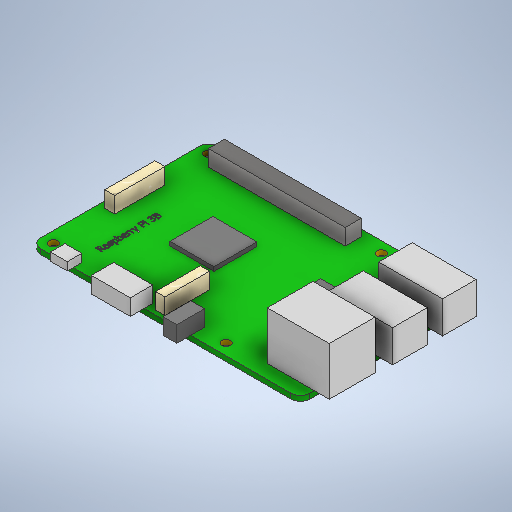
# Autodesk Inventor part: RPi3B
Saved by Autodesk Inventor 2025 (Build 290162000, 162)
## iProperties
Created: 2025-05-10
Part Number: RPi3B
Material: Generic
Document SubType Name: Modeling
Designer: thesn
Density: 1 g/cm^3
Appearance: Default
Author: thesn
Autodesk Inventor part; units mm, degrees
ref_plane "YZ Plane" through (0, 0, 0) normal (1, 0, 0) x (0, 1, 0)
ref_plane "XZ Plane" through (0, 0, 0) normal (0, 1, 0) x (-1, 0, 0)
ref_plane "XY Plane" through (0, 0, 0) normal (0, 0, 1) x (1, 0, 0)
sketch "Sketch1" plane through (0, 0, 0) normal (0, 1, 0) x (-1, 0, 0)
  line L0 (0, 0) -> (-85.0001, 0)
  line L1 (-85.0001, 0) -> (-85.0001, -55.9999)
  line L2 (-85.0001, -55.9999) -> (0, -55.9999)
  line L3 (0, -55.9999) -> (0, 0)
  dimension "d0" = 85.0001
  dimension "d1" = 55.9999
  constraints: 8 end point, 2 parallel, 1 horizontal, 1 perpendicular
  measures "d0" distance of L2.end L1.end
  measures "d1" distance of L1.end L0.end
extrude "Extrusion1" add sketch "Sketch1" along normal blind 1.6
fillet "Fillet1" radius 3 4 edges at (0, 0.8, -55.9999) (85.0001, 0.8, -55.9999) (0, 0.8, 0) (85.0001, 0.8, 0)
sketch "Sketch2" plane through (0, 1.6, 0) normal (0, 1, 0) x (1, 0, 0)
  circle A0 centre (3.5, 3.5) radius 1.375
  line L0 (3, 0) -> (82.0001, 0) projected
  line L1 (0, 52.9999) -> (0, 3) projected
  circle A1 centre (3.5, 52.4999) radius 1.375
  circle A2 centre (58.0001, 52.4999) radius 1.375
  circle A3 centre (58.0001, 3.5) radius 1.375
  line L2 (82.0001, 55.9999) -> (3, 55.9999) projected
  line L3 (85.0001, 3) -> (85.0001, 52.9999) projected
  point P0 (0, 0)
  dimension "d5" = 2.75
  dimension "d6" = 3.5
  dimension "d7" = 3.5
  dimension "d10" = 2.75
  dimension "d11" = 2.75
  dimension "d12" = 2.75
  dimension "d13" = 3.5
  dimension "d14" = 3.5
  dimension "d15" = 3.5
  dimension "d16" = 3.5
  dimension "d17" = 26.9999
  dimension "d18" = 26.9999
  constraints: 4 centre point
  measures "d5" diameter of A0
  measures "d6" distance from line of L0 A0.centre
  measures "d7" distance from line of L1 A0.centre
  measures "d10" diameter of A1
  measures "d11" diameter of A2
  measures "d12" diameter of A3
  measures "d13" distance from line of L1 A1.centre
  measures "d14" distance from line of L2 A1.centre
  measures "d15" distance from line of L2 A2.centre
  measures "d16" distance from line of L0 A3.centre
  measures "d17" distance from line of L3 A2.centre
  measures "d18" distance from line of L3 A3.centre
extrude "Extrusion2" cut sketch "Sketch2" against normal blind 25.4
sketch "Sketch3" plane through (0, 1.6, 0) normal (0, 1, 0) x (1, 0, 0)
  line L0 (7.1379, 53.8738) -> (50.3179, 53.8738)
  line L1 (50.3179, 53.8738) -> (50.3179, 48.7938)
  line L2 (50.3179, 48.7938) -> (7.1379, 48.7938)
  line L3 (7.1379, 48.7938) -> (7.1379, 53.8738)
  line L4 (70.1256, 50.1514) -> (90.2699, 50.1514)
  line L5 (90.2699, 50.1514) -> (90.2699, 39.5684)
  line L6 (90.2699, 39.5684) -> (70.1256, 39.5684)
  line L7 (70.1256, 39.5684) -> (70.1256, 50.1514)
  line L8 (70.1256, 34.7512) -> (90.2699, 34.7512)
  line L9 (90.2699, 34.7512) -> (90.2699, 23.8032)
  line L10 (90.2699, 23.8032) -> (70.1256, 23.8032)
  line L11 (70.1256, 23.8032) -> (70.1256, 34.7512)
  line L12 (70.1256, 18.8401) -> (89.686, 18.8401)
  line L13 (89.686, 18.8401) -> (89.686, 4.3887)
  line L14 (89.686, 4.3887) -> (70.1256, 4.3887)
  line L15 (70.1256, 4.3887) -> (70.1256, 18.8401)
  line L16 (7.9408, 2.71) -> (13.2688, 2.71)
  line L17 (13.2688, 2.71) -> (13.2688, -1.8882)
  line L18 (13.2688, -1.8882) -> (7.9408, -1.8882)
  line L19 (7.9408, -1.8882) -> (7.9408, 2.71)
  line L20 (23.3149, 2.71) -> (35.6326, 2.71)
  line L21 (35.6326, 2.71) -> (35.6326, -4.3596)
  line L22 (35.6326, -4.3596) -> (23.3149, -4.3596)
  line L23 (23.3149, -4.3596) -> (23.3149, 2.71)
  line L24 (45.9794, 4.3887) -> (50.3179, 4.3887)
  line L25 (50.3179, 4.3887) -> (50.3179, -4.3596)
  line L26 (50.3179, -4.3596) -> (45.9794, -4.3596)
  line L27 (45.9794, -4.3596) -> (45.9794, 4.3887)
  line L28 (2.0299, 37.0278) -> (5.1833, 37.0278)
  line L29 (5.1833, 37.0278) -> (5.1833, 21.1626)
  line L30 (5.1833, 21.1626) -> (2.0299, 21.1626)
  line L31 (2.0299, 21.1626) -> (2.0299, 37.0278)
  line L32 (22.6251, 34.7512) -> (36.5195, 34.7512)
  line L33 (36.5195, 34.7512) -> (36.5195, 21.1626)
  line L34 (36.5195, 21.1626) -> (22.6251, 21.1626)
  line L35 (22.6251, 21.1626) -> (22.6251, 34.7512)
  line L36 (56.6219, 34.7512) -> (65.4907, 34.7512)
  line L37 (65.4907, 34.7512) -> (65.4907, 26.0897)
  line L38 (65.4907, 26.0897) -> (56.6219, 26.0897)
  line L39 (56.6219, 26.0897) -> (56.6219, 34.7512)
  line L40 (37.899, 15.4472) -> (40.8553, 15.4472)
  line L41 (40.8553, 15.4472) -> (40.8553, 1.3558)
  line L42 (40.8553, 1.3558) -> (37.899, 1.3558)
  line L43 (37.899, 1.3558) -> (37.899, 15.4472)
  point P0 (0, 0)
  dimension "d19" = 43.18
  dimension "d20" = 5.08
  constraints: 88 end point, 22 parallel, 11 horizontal, 11 perpendicular, 9 point on line
  measures "d19" distance of L1.end L2.end
  measures "d20" distance of L0.end L1.end
extrude "Extrusion3" add sketch "Sketch3" along normal blind 10.16 contours L4 L5 L6 L7 | L8 L9 L10 L11
extrude "Extrusion4" add sketch "Sketch3" along normal blind 15.24 contours L12 L13 L14 L15
extrude "Extrusion5" add sketch "Sketch3" along normal blind 5.08 contours L0 L1 L2 L3
extrude "Extrusion6" add sketch "Sketch3" along normal blind 1.27 contours L32 L33 L34 L35 | L36 L37 L38 L39
extrude "Extrusion7" add sketch "Sketch3" along normal blind 5.08 contours L28 L29 L30 L31 | L40 L41 L42 L43
extrude "Extrusion8" add sketch "Sketch3" along normal blind 5.08 contours L20 L21 L22 L23
extrude "Extrusion9" add sketch "Sketch3" along normal blind 2.54 contours L16 L17 L18 L19
extrude "Extrusion10" add sketch "Sketch3" along normal blind 5.08 contours L24 L25 L26 L27
sketch "Sketch4" plane through (0, 0, 0) normal (0, -1, 0) x (1, 0, 0)
  line L0 (28.4319, -19.6331) -> (43.4029, -19.6331)
  line L1 (43.4029, -19.6331) -> (43.4029, -33.6849)
  line L2 (43.4029, -33.6849) -> (28.4319, -33.6849)
  line L3 (28.4319, -33.6849) -> (28.4319, -19.6331)
  line L4 (0.8536, -19.6331) -> (8.7331, -19.6331)
  line L5 (8.7331, -19.6331) -> (8.7331, -30.2704)
  line L6 (8.7331, -30.2704) -> (0.8536, -30.2704)
  line L7 (0.8536, -30.2704) -> (0.8536, -19.6331)
  point P0 (0, 0)
  constraints: 16 end point, 4 parallel, 2 horizontal, 2 perpendicular, 1 point on line
extrude "Extrusion11" add sketch "Sketch4" along normal blind 1.27 contours L0 L1 L2 L3
extrude "Extrusion12" add sketch "Sketch4" along normal blind 0.508 contours L4 L5 L6 L7
sketch "Sketch5" plane through (0, 1.6, 0) normal (0, 1, 0) x (1, 0, 0)
  line L0 (11.2333, 8.619) -> (11.2333, 37.8862) construction
  line L1 (11.2333, 37.8862) -> (15.2594, 37.8862) construction
  line L2 (15.2594, 37.8862) -> (15.2594, 8.619) construction
  line L3 (15.2594, 8.619) -> (11.2333, 8.619) construction
  line L4 (13.3559, 10.3974) -> (13.3559, 10.0467)
  line L5 (13.3559, 10.0467) -> (12.5474, 9.4045)
  line L6 (12.5474, 9.4045) -> (12.5474, 9.0949)
  line L7 (12.5474, 9.0949) -> (13.3559, 9.0949)
  line L8 (13.3559, 9.0949) -> (13.3559, 8.8249)
  line L9 (13.3559, 8.8249) -> (11.3239, 8.8249)
  line L10 (11.3239, 8.8249) -> (11.3239, 9.3485)
  spline S0 degree 2 poles (11.3239, 9.3485) (11.3239, 9.523) (11.3618, 9.7585) (11.4309, 9.8656) knots 0 0 0 1 2 2 2
  spline S1 degree 2 poles (11.4309, 9.8656) (11.5001, 9.9726) (11.7158, 10.0961) (11.8755, 10.0961) knots 0 0 0 1 2 2 2
  spline S2 degree 2 poles (11.8755, 10.0961) (12.0978, 10.0961) (12.3992, 9.8688) (12.4716, 9.6745) knots 0 0 0 1 2 2 2
  line L11 (12.4716, 9.6745) -> (13.3559, 10.3974)
  spline S3 degree 2 poles (11.8969, 9.8145) (11.808, 9.8145) (11.6713, 9.7519) (11.6269, 9.6861) knots 0 0 0 1 2 2 2
  spline S4 degree 2 poles (11.6269, 9.6861) (11.589, 9.6284) (11.5577, 9.4753) (11.5577, 9.3633) knots 0 0 0 1 2 2 2
  line L12 (11.5577, 9.3633) -> (11.5577, 9.0949)
  line L13 (11.5577, 9.0949) -> (12.3218, 9.0949)
  line L14 (12.3218, 9.0949) -> (12.3218, 9.332)
  spline S5 degree 2 poles (12.3218, 9.332) (12.3218, 9.4489) (12.2806, 9.635) (12.2164, 9.6992) knots 0 0 0 1 2 2 2
  spline S6 degree 2 poles (12.2164, 9.6992) (12.1604, 9.7585) (12.0023, 9.8145) (11.8969, 9.8145) knots 0 0 0 1 2 2 2
  spline S7 degree 2 poles (13.1945, 11.3887) (13.2176, 11.3574) (13.2999, 11.2521) (13.3246, 11.2027) knots 0 0 0 1 2 2 2
  spline S8 degree 2 poles (13.3246, 11.2027) (13.3608, 11.1351) (13.3987, 11.0083) (13.3987, 10.8931) knots 0 0 0 1 2 2 2
  spline S9 degree 2 poles (13.3987, 10.8931) (13.3987, 10.7992) (13.3279, 10.6296) (13.2637, 10.5654) knots 0 0 0 1 2 2 2
  spline S10 degree 2 poles (13.2637, 10.5654) (13.2011, 10.5045) (13.0167, 10.4304) (12.9146, 10.4304) knots 0 0 0 1 2 2 2
  spline S11 degree 2 poles (12.9146, 10.4304) (12.7565, 10.4304) (12.5325, 10.5637) (12.4683, 10.7087) knots 0 0 0 1 2 2 2
  spline S12 degree 2 poles (12.4683, 10.7087) (12.409, 10.8371) (12.3646, 11.1862) (12.3531, 11.3887) knots 0 0 0 1 2 2 2
  line L15 (12.3531, 11.3887) -> (12.3037, 11.3887)
  spline S13 degree 2 poles (12.3037, 11.3887) (12.2147, 11.3887) (12.1044, 11.3344) (12.0731, 11.285) knots 0 0 0 1 2 2 2
  spline S14 degree 2 poles (12.0731, 11.285) (12.0418, 11.2356) (12.0221, 11.094) (12.0221, 11.0182) knots 0 0 0 1 2 2 2
  spline S15 degree 2 poles (12.0221, 11.0182) (12.0221, 10.9293) (12.0748, 10.6889) (12.1258, 10.5687) knots 0 0 0 1 2 2 2
  line L16 (12.1258, 10.5687) -> (12.1258, 10.5539)
  line L17 (12.1258, 10.5539) -> (11.864, 10.5539)
  spline S16 degree 2 poles (11.864, 10.5539) (11.8442, 10.6247) (11.7948, 10.8898) (11.7948, 11.0199) knots 0 0 0 1 2 2 2
  spline S17 degree 2 poles (11.7948, 11.0199) (11.7948, 11.178) (11.8442, 11.3937) (11.9085, 11.4793) knots 0 0 0 1 2 2 2
  spline S18 degree 2 poles (11.9085, 11.4793) (11.971, 11.5633) (12.1703, 11.6456) (12.3135, 11.6456) knots 0 0 0 1 2 2 2
  line L18 (12.3135, 11.6456) -> (13.3559, 11.6456)
  line L19 (13.3559, 11.6456) -> (13.3559, 11.3887)
  line L20 (13.3559, 11.3887) -> (13.1945, 11.3887)
  line L21 (12.9804, 11.3887) -> (12.5572, 11.3887)
  spline S19 degree 2 poles (12.5572, 11.3887) (12.5655, 11.2965) (12.5935, 11.0182) (12.6198, 10.931) knots 0 0 0 1 2 2 2
  spline S20 degree 2 poles (12.6198, 10.931) (12.6511, 10.8289) (12.7812, 10.6955) (12.8965, 10.6955) knots 0 0 0 1 2 2 2
  spline S21 degree 2 poles (12.8965, 10.6955) (13.0282, 10.6955) (13.1616, 10.8437) (13.1616, 10.9853) knots 0 0 0 1 2 2 2
  spline S22 degree 2 poles (13.1616, 10.9853) (13.1616, 11.1055) (13.0578, 11.3031) (12.9804, 11.3887) knots 0 0 0 1 2 2 2
  spline S23 degree 2 poles (13.3921, 12.4179) (13.3921, 12.2648) (13.3098, 11.9996) (13.2637, 11.9124) knots 0 0 0 1 2 2 2
  line L22 (13.2637, 11.9124) -> (12.9755, 11.9124)
  line L23 (12.9755, 11.9124) -> (12.9755, 11.9255)
  spline S24 degree 2 poles (12.9755, 11.9255) (13.0019, 11.9585) (13.0644, 12.0474) (13.099, 12.1215) knots 0 0 0 1 2 2 2
  spline S25 degree 2 poles (13.099, 12.1215) (13.1303, 12.1857) (13.1764, 12.3438) (13.1764, 12.4278) knots 0 0 0 1 2 2 2
  spline S26 degree 2 poles (13.1764, 12.4278) (13.1764, 12.4887) (13.1484, 12.6287) (13.1254, 12.6616) knots 0 0 0 1 2 2 2
  spline S27 degree 2 poles (13.1254, 12.6616) (13.0941, 12.7094) (13.0233, 12.7522) (12.9508, 12.7522) knots 0 0 0 1 2 2 2
  spline S28 degree 2 poles (12.9508, 12.7522) (12.8602, 12.7522) (12.7664, 12.6534) (12.7351, 12.5266) knots 0 0 0 1 2 2 2
  spline S29 degree 2 poles (12.7351, 12.5266) (12.7236, 12.4772) (12.6906, 12.3191) (12.6725, 12.2516) knots 0 0 0 1 2 2 2
  spline S30 degree 2 poles (12.6725, 12.2516) (12.6215, 12.077) (12.4107, 11.919) (12.2608, 11.919) knots 0 0 0 1 2 2 2
  spline S31 degree 2 poles (12.2608, 11.919) (12.0534, 11.919) (11.7948, 12.2302) (11.7948, 12.4871) knots 0 0 0 1 2 2 2
  spline S32 degree 2 poles (11.7948, 12.4871) (11.7948, 12.6139) (11.8574, 12.8707) (11.9052, 12.958) knots 0 0 0 1 2 2 2
  line L24 (11.9052, 12.958) -> (12.1802, 12.958)
  line L25 (12.1802, 12.958) -> (12.1802, 12.9448)
  spline S33 degree 2 poles (12.1802, 12.9448) (12.1011, 12.846) (12.0106, 12.6056) (12.0106, 12.4821) knots 0 0 0 1 2 2 2
  spline S34 degree 2 poles (12.0106, 12.4821) (12.0106, 12.3553) (12.1176, 12.1808) (12.2246, 12.1808) knots 0 0 0 1 2 2 2
  spline S35 degree 2 poles (12.2246, 12.1808) (12.3218, 12.1808) (12.4156, 12.2845) (12.4453, 12.3998) knots 0 0 0 1 2 2 2
  spline S36 degree 2 poles (12.4453, 12.3998) (12.4601, 12.4558) (12.4897, 12.5974) (12.5078, 12.6748) knots 0 0 0 1 2 2 2
  spline S37 degree 2 poles (12.5078, 12.6748) (12.5507, 12.8427) (12.7466, 13.014) (12.9162, 13.014) knots 0 0 0 1 2 2 2
  spline S38 degree 2 poles (12.9162, 13.014) (13.015, 13.014) (13.1896, 12.9366) (13.2538, 12.8609) knots 0 0 0 1 2 2 2
  spline S39 degree 2 poles (13.2538, 12.8609) (13.3213, 12.7802) (13.3921, 12.5743) (13.3921, 12.4179) knots 0 0 0 1 2 2 2
  spline S40 degree 2 poles (12.5523, 14.5306) (12.9343, 14.5306) (13.3855, 14.1667) (13.3855, 13.8884) knots 0 0 0 1 2 2 2
  spline S41 degree 2 poles (13.3855, 13.8884) (13.3855, 13.7748) (13.3328, 13.6002) (13.2785, 13.5097) knots 0 0 0 1 2 2 2
  line L26 (13.2785, 13.5097) -> (13.9174, 13.5097)
  line L27 (13.9174, 13.5097) -> (13.9174, 13.2528)
  line L28 (13.9174, 13.2528) -> (11.8311, 13.2528)
  line L29 (11.8311, 13.2528) -> (11.8311, 13.5097)
  line L30 (11.8311, 13.5097) -> (11.9908, 13.5097)
  spline S42 degree 2 poles (11.9908, 13.5097) (11.9035, 13.6052) (11.7882, 13.839) (11.7882, 13.9757) knots 0 0 0 1 2 2 2
  spline S43 degree 2 poles (11.7882, 13.9757) (11.7882, 14.2375) (12.2032, 14.5306) (12.5523, 14.5306) knots 0 0 0 1 2 2 2
  spline S44 degree 2 poles (12.5819, 14.2655) (12.3201, 14.2655) (12.032, 14.0992) (12.032, 13.9131) knots 0 0 0 1 2 2 2
  spline S45 degree 2 poles (12.032, 13.9131) (12.032, 13.8044) (12.1291, 13.6002) (12.2049, 13.5097) knots 0 0 0 1 2 2 2
  line L31 (12.2049, 13.5097) -> (13.071, 13.5097)
  spline S46 degree 2 poles (13.071, 13.5097) (13.1188, 13.6101) (13.155, 13.7534) (13.155, 13.8456) knots 0 0 0 1 2 2 2
  spline S47 degree 2 poles (13.155, 13.8456) (13.155, 14.0448) (12.8619, 14.2655) (12.5819, 14.2655) knots 0 0 0 1 2 2 2
  spline S48 degree 2 poles (12.5688, 16.0752) (12.9426, 16.0752) (13.3987, 15.7129) (13.3987, 15.4396) knots 0 0 0 1 2 2 2
  spline S49 degree 2 poles (13.3987, 15.4396) (13.3987, 15.3161) (13.3378, 15.1399) (13.2851, 15.0542) knots 0 0 0 1 2 2 2
  line L32 (13.2851, 15.0542) -> (13.3559, 15.0378)
  line L33 (13.3559, 15.0378) -> (13.3559, 14.7974)
  line L34 (13.3559, 14.7974) -> (11.2333, 14.7974)
  line L35 (11.2333, 14.7974) -> (11.2333, 15.0542)
  line L36 (11.2333, 15.0542) -> (11.9908, 15.0542)
  spline S50 degree 2 poles (11.9908, 15.0542) (11.9035, 15.1514) (11.7882, 15.377) (11.7882, 15.5202) knots 0 0 0 1 2 2 2
  spline S51 degree 2 poles (11.7882, 15.5202) (11.7882, 15.7788) (12.2016, 16.0752) (12.5688, 16.0752) knots 0 0 0 1 2 2 2
  spline S52 degree 2 poles (12.5885, 15.8101) (12.3152, 15.8101) (12.032, 15.6437) (12.032, 15.4593) knots 0 0 0 1 2 2 2
  spline S53 degree 2 poles (12.032, 15.4593) (12.032, 15.3556) (12.1308, 15.1415) (12.2065, 15.0542) knots 0 0 0 1 2 2 2
  line L37 (12.2065, 15.0542) -> (13.0809, 15.0542)
  spline S54 degree 2 poles (13.0809, 15.0542) (13.1286, 15.1514) (13.1682, 15.3012) (13.1682, 15.3902) knots 0 0 0 1 2 2 2
  spline S55 degree 2 poles (13.1682, 15.3902) (13.1682, 15.5861) (12.8899, 15.8101) (12.5885, 15.8101) knots 0 0 0 1 2 2 2
  spline S56 degree 2 poles (13.3905, 17.0039) (13.3905, 16.6383) (12.9804, 16.2366) (12.6017, 16.2366) knots 0 0 0 1 2 2 2
  spline S57 degree 2 poles (12.6017, 16.2366) (12.2296, 16.2366) (11.7882, 16.6268) (11.7882, 16.9413) knots 0 0 0 1 2 2 2
  spline S58 degree 2 poles (11.7882, 16.9413) (11.7882, 17.0829) (11.8706, 17.302) (11.9579, 17.3826) knots 0 0 0 1 2 2 2
  spline S59 degree 2 poles (11.9579, 17.3826) (12.0451, 17.465) (12.2971, 17.5522) (12.4799, 17.5522) knots 0 0 0 1 2 2 2
  line L38 (12.4799, 17.5522) -> (12.6198, 17.5522)
  line L39 (12.6198, 17.5522) -> (12.6198, 16.4967)
  spline S60 degree 2 poles (12.6198, 16.4967) (12.8849, 16.4967) (13.1665, 16.7635) (13.1665, 17.0006) knots 0 0 0 1 2 2 2
  spline S61 degree 2 poles (13.1665, 17.0006) (13.1665, 17.0846) (13.1286, 17.2476) (13.099, 17.3135) knots 0 0 0 1 2 2 2
  spline S62 degree 2 poles (13.099, 17.3135) (13.0661, 17.3826) (13.0084, 17.4781) (12.9821, 17.5094) knots 0 0 0 1 2 2 2
  line L40 (12.9821, 17.5094) -> (12.9821, 17.5243)
  line L41 (12.9821, 17.5243) -> (13.262, 17.5243)
  spline S63 degree 2 poles (13.262, 17.5243) (13.2801, 17.4798) (13.3328, 17.3448) (13.3477, 17.2921) knots 0 0 0 1 2 2 2
  spline S64 degree 2 poles (13.3477, 17.2921) (13.3691, 17.218) (13.3905, 17.0961) (13.3905, 17.0039) knots 0 0 0 1 2 2 2
  spline S65 degree 2 poles (12.4239, 17.302) (12.3201, 17.2987) (12.1686, 17.2558) (12.1176, 17.2147) knots 0 0 0 1 2 2 2
  spline S66 degree 2 poles (12.1176, 17.2147) (12.06, 17.1702) (11.999, 17.0302) (11.999, 16.9265) knots 0 0 0 1 2 2 2
  spline S67 degree 2 poles (11.999, 16.9265) (11.999, 16.8244) (12.06, 16.6812) (12.1192, 16.6219) knots 0 0 0 1 2 2 2
  spline S68 degree 2 poles (12.1192, 16.6219) (12.1802, 16.5642) (12.3267, 16.505) (12.4239, 16.4967) knots 0 0 0 1 2 2 2
  line L42 (12.4239, 16.4967) -> (12.4239, 17.302)
  line L43 (12.1061, 18.6209) -> (12.1061, 18.6078)
  spline S69 degree 2 poles (12.1061, 18.6078) (12.0978, 18.5781) (12.0945, 18.5139) (12.0945, 18.4694) knots 0 0 0 1 2 2 2
  spline S70 degree 2 poles (12.0945, 18.4694) (12.0945, 18.3657) (12.1851, 18.1615) (12.274, 18.0693) knots 0 0 0 1 2 2 2
  line L44 (12.274, 18.0693) -> (13.3559, 18.0693)
  line L45 (13.3559, 18.0693) -> (13.3559, 17.8124)
  line L46 (13.3559, 17.8124) -> (11.8311, 17.8124)
  line L47 (11.8311, 17.8124) -> (11.8311, 18.0693)
  line L48 (11.8311, 18.0693) -> (12.0583, 18.0693)
  spline S71 degree 2 poles (12.0583, 18.0693) (11.9332, 18.2093) (11.8311, 18.4184) (11.8311, 18.5172) knots 0 0 0 1 2 2 2
  spline S72 degree 2 poles (11.8311, 18.5172) (11.8311, 18.5567) (11.8344, 18.5962) (11.8393, 18.6209) knots 0 0 0 1 2 2 2
  line L49 (11.8393, 18.6209) -> (12.1061, 18.6209)
  line L50 (12.1061, 19.6287) -> (12.1061, 19.6155)
  spline S73 degree 2 poles (12.1061, 19.6155) (12.0978, 19.5859) (12.0945, 19.5217) (12.0945, 19.4772) knots 0 0 0 1 2 2 2
  spline S74 degree 2 poles (12.0945, 19.4772) (12.0945, 19.3735) (12.1851, 19.1693) (12.274, 19.0771) knots 0 0 0 1 2 2 2
  line L51 (12.274, 19.0771) -> (13.3559, 19.0771)
  line L52 (13.3559, 19.0771) -> (13.3559, 18.8202)
  line L53 (13.3559, 18.8202) -> (11.8311, 18.8202)
  line L54 (11.8311, 18.8202) -> (11.8311, 19.0771)
  line L55 (11.8311, 19.0771) -> (12.0583, 19.0771)
  spline S75 degree 2 poles (12.0583, 19.0771) (11.9332, 19.217) (11.8311, 19.4262) (11.8311, 19.525) knots 0 0 0 1 2 2 2
  spline S76 degree 2 poles (11.8311, 19.525) (11.8311, 19.5645) (11.8344, 19.604) (11.8393, 19.6287) knots 0 0 0 1 2 2 2
  line L56 (11.8393, 19.6287) -> (12.1061, 19.6287)
  line L57 (11.8311, 21.0251) -> (13.9174, 20.205)
  line L58 (13.9174, 20.205) -> (13.9174, 19.93)
  line L59 (13.9174, 19.93) -> (13.2818, 20.2034)
  line L60 (13.2818, 20.2034) -> (11.8311, 19.6501)
  line L61 (11.8311, 19.6501) -> (11.8311, 19.9268)
  line L62 (11.8311, 19.9268) -> (12.9607, 20.3434)
  line L63 (12.9607, 20.3434) -> (11.8311, 20.7583)
  line L64 (11.8311, 20.7583) -> (11.8311, 21.0251)
  spline S77 degree 2 poles (11.9365, 23.3963) (12.0682, 23.3963) (12.3053, 23.3024) (12.3876, 23.2185) knots 0 0 0 1 2 2 2
  spline S78 degree 2 poles (12.3876, 23.2185) (12.4914, 23.1131) (12.5984, 22.8282) (12.5984, 22.6108) knots 0 0 0 1 2 2 2
  line L65 (12.5984, 22.6108) -> (12.5984, 22.382)
  line L66 (12.5984, 22.382) -> (13.3559, 22.382)
  line L67 (13.3559, 22.382) -> (13.3559, 22.1119)
  line L68 (13.3559, 22.1119) -> (11.3239, 22.1119)
  line L69 (11.3239, 22.1119) -> (11.3239, 22.6224)
  spline S79 degree 2 poles (11.3239, 22.6224) (11.3239, 22.8035) (11.3832, 23.0571) (11.4507, 23.1542) knots 0 0 0 1 2 2 2
  spline S80 degree 2 poles (11.4507, 23.1542) (11.5281, 23.2679) (11.7668, 23.3963) (11.9365, 23.3963) knots 0 0 0 1 2 2 2
  spline S81 degree 2 poles (11.9447, 23.1147) (11.8393, 23.1147) (11.6845, 23.0423) (11.6351, 22.9682) knots 0 0 0 1 2 2 2
  spline S82 degree 2 poles (11.6351, 22.9682) (11.5923, 22.9039) (11.5577, 22.7327) (11.5577, 22.6059) knots 0 0 0 1 2 2 2
  line L70 (11.5577, 22.6059) -> (11.5577, 22.382)
  line L71 (11.5577, 22.382) -> (12.3679, 22.382)
  line L72 (12.3679, 22.382) -> (12.3679, 22.5664)
  spline S83 degree 2 poles (12.3679, 22.5664) (12.3679, 22.731) (12.3152, 22.9336) (12.246, 22.9995) knots 0 0 0 1 2 2 2
  spline S84 degree 2 poles (12.246, 22.9995) (12.1851, 23.0604) (12.0418, 23.1147) (11.9447, 23.1147) knots 0 0 0 1 2 2 2
  line L73 (13.3559, 23.8952) -> (13.3559, 23.6384)
  line L74 (13.3559, 23.6384) -> (11.8311, 23.6384)
  line L75 (11.8311, 23.6384) -> (11.8311, 23.8952)
  line L76 (11.8311, 23.8952) -> (13.3559, 23.8952)
  line L77 (11.5775, 23.9134) -> (11.5775, 23.6219)
  line L78 (11.5775, 23.6219) -> (11.3107, 23.6219)
  line L79 (11.3107, 23.6219) -> (11.3107, 23.9134)
  line L80 (11.3107, 23.9134) -> (11.5775, 23.9134)
  spline S85 degree 2 poles (11.5165, 25.6555) (11.5165, 25.5814) (11.5528, 25.4349) (11.5808, 25.3641) knots 0 0 0 1 2 2 2
  spline S86 degree 2 poles (11.5808, 25.3641) (11.6088, 25.2982) (11.668, 25.2011) (11.6944, 25.1632) knots 0 0 0 1 2 2 2
  line L81 (11.6944, 25.1632) -> (11.6944, 25.1467)
  line L82 (11.6944, 25.1467) -> (11.4062, 25.1467)
  spline S87 degree 2 poles (11.4062, 25.1467) (11.3585, 25.2356) (11.2811, 25.5403) (11.2811, 25.677) knots 0 0 0 1 2 2 2
  spline S88 degree 2 poles (11.2811, 25.677) (11.2811, 25.8153) (11.3371, 26.0211) (11.3963, 26.1051) knots 0 0 0 1 2 2 2
  spline S89 degree 2 poles (11.3963, 26.1051) (11.4606, 26.194) (11.6466, 26.2862) (11.7718, 26.2862) knots 0 0 0 1 2 2 2
  spline S90 degree 2 poles (11.7718, 26.2862) (11.9397, 26.2862) (12.1933, 26.0656) (12.2263, 25.9108) knots 0 0 0 1 2 2 2
  line L83 (12.2263, 25.9108) -> (12.246, 25.9108)
  spline S91 degree 2 poles (12.246, 25.9108) (12.2592, 25.975) (12.3185, 26.1216) (12.3778, 26.1841) knots 0 0 0 1 2 2 2
  spline S92 degree 2 poles (12.3778, 26.1841) (12.4354, 26.2467) (12.6198, 26.3257) (12.7532, 26.3257) knots 0 0 0 1 2 2 2
  spline S93 degree 2 poles (12.7532, 26.3257) (12.8899, 26.3257) (13.1221, 26.2319) (13.211, 26.1463) knots 0 0 0 1 2 2 2
  spline S94 degree 2 poles (13.211, 26.1463) (13.3032, 26.0573) (13.3987, 25.8054) (13.3987, 25.6457) knots 0 0 0 1 2 2 2
  spline S95 degree 2 poles (13.3987, 25.6457) (13.3987, 25.4925) (13.3246, 25.1928) (13.2736, 25.0907) knots 0 0 0 1 2 2 2
  line L84 (13.2736, 25.0907) -> (12.9854, 25.0907)
  line L85 (12.9854, 25.0907) -> (12.9854, 25.1105)
  spline S96 degree 2 poles (12.9854, 25.1105) (13.048, 25.1961) (13.1632, 25.4859) (13.1632, 25.6292) knots 0 0 0 1 2 2 2
  spline S97 degree 2 poles (13.1632, 25.6292) (13.1632, 25.7132) (13.1105, 25.8811) (13.0496, 25.9371) knots 0 0 0 1 2 2 2
  spline S98 degree 2 poles (13.0496, 25.9371) (12.9887, 25.9915) (12.8438, 26.0491) (12.7334, 26.0491) knots 0 0 0 1 2 2 2
  spline S99 degree 2 poles (12.7334, 26.0491) (12.6231, 26.0491) (12.4799, 25.9849) (12.4387, 25.9272) knots 0 0 0 1 2 2 2
  spline S100 degree 2 poles (12.4387, 25.9272) (12.3975, 25.8696) (12.3662, 25.7132) (12.3662, 25.621) knots 0 0 0 1 2 2 2
  line L86 (12.3662, 25.621) -> (12.3662, 25.5057)
  line L87 (12.3662, 25.5057) -> (12.1406, 25.5057)
  line L88 (12.1406, 25.5057) -> (12.1406, 25.5963)
  spline S101 degree 2 poles (12.1406, 25.5963) (12.1406, 25.779) (11.9661, 26.0096) (11.7998, 26.0096) knots 0 0 0 1 2 2 2
  spline S102 degree 2 poles (11.7998, 26.0096) (11.7224, 26.0096) (11.6121, 25.9503) (11.5791, 25.9025) knots 0 0 0 1 2 2 2
  spline S103 degree 2 poles (11.5791, 25.9025) (11.5445, 25.8515) (11.5165, 25.7264) (11.5165, 25.6555) knots 0 0 0 1 2 2 2
  spline S104 degree 2 poles (12.7318, 28.0679) (12.8833, 28.0679) (13.1155, 27.9527) (13.1912, 27.8572) knots 0 0 0 1 2 2 2
  spline S105 degree 2 poles (13.1912, 27.8572) (13.2801, 27.7419) (13.3559, 27.4801) (13.3559, 27.2726) knots 0 0 0 1 2 2 2
  line L89 (13.3559, 27.2726) -> (13.3559, 26.6897)
  line L90 (13.3559, 26.6897) -> (11.3239, 26.6897)
  line L91 (11.3239, 26.6897) -> (11.3239, 27.2281)
  spline S106 degree 2 poles (11.3239, 27.2281) (11.3239, 27.4455) (11.3519, 27.6628) (11.4062, 27.7616) knots 0 0 0 1 2 2 2
  spline S107 degree 2 poles (11.4062, 27.7616) (11.4639, 27.872) (11.6532, 27.9724) (11.7817, 27.9724) knots 0 0 0 1 2 2 2
  spline S108 degree 2 poles (11.7817, 27.9724) (11.9249, 27.9724) (12.1522, 27.8209) (12.2164, 27.6875) knots 0 0 0 1 2 2 2
  line L92 (12.2164, 27.6875) -> (12.2263, 27.6875)
  spline S109 degree 2 poles (12.2263, 27.6875) (12.2757, 27.8687) (12.5375, 28.0679) (12.7318, 28.0679) knots 0 0 0 1 2 2 2
  spline S110 degree 2 poles (12.7433, 27.7863) (12.6281, 27.7863) (12.4799, 27.7205) (12.4272, 27.6217) knots 0 0 0 1 2 2 2
  spline S111 degree 2 poles (12.4272, 27.6217) (12.3942, 27.5575) (12.3745, 27.406) (12.3745, 27.266) knots 0 0 0 1 2 2 2
  line L93 (12.3745, 27.266) -> (12.3745, 26.9597)
  line L94 (12.3745, 26.9597) -> (13.1254, 26.9597)
  line L95 (13.1254, 26.9597) -> (13.1254, 27.1787)
  spline S112 degree 2 poles (13.1254, 27.1787) (13.1254, 27.3566) (13.0924, 27.5608) (13.0397, 27.6398) knots 0 0 0 1 2 2 2
  spline S113 degree 2 poles (13.0397, 27.6398) (12.9854, 27.7155) (12.8504, 27.7863) (12.7433, 27.7863) knots 0 0 0 1 2 2 2
  spline S114 degree 2 poles (11.8195, 27.6908) (11.7471, 27.6908) (11.6384, 27.6414) (11.6071, 27.5871) knots 0 0 0 1 2 2 2
  spline S115 degree 2 poles (11.6071, 27.5871) (11.5709, 27.5212) (11.5544, 27.3615) (11.5544, 27.2182) knots 0 0 0 1 2 2 2
  line L96 (11.5544, 27.2182) -> (11.5544, 26.9597)
  line L97 (11.5544, 26.9597) -> (12.1489, 26.9597)
  line L98 (12.1489, 26.9597) -> (12.1489, 27.266)
  spline S116 degree 2 poles (12.1489, 27.266) (12.1489, 27.3928) (12.1225, 27.513) (12.0814, 27.5772) knots 0 0 0 1 2 2 2
  spline S117 degree 2 poles (12.0814, 27.5772) (12.0418, 27.6398) (11.915, 27.6908) (11.8195, 27.6908) knots 0 0 0 1 2 2 2
  point P0 (0, 0)
  constraints: 2 other
extrude "Extrusion13" cut sketch "Sketch5" against normal blind 0.508
body "Solid1"
